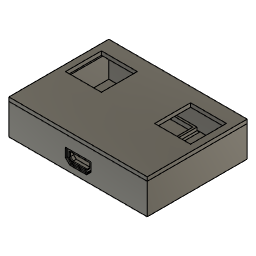
keypad_choc_white_1kgap (Autodesk Fusion 360 design; units mm, degrees)
Autodesk Fusion 360 part; units mm, degrees
sketch "Sketch1" plane through (0, 0, 0) normal (0, 0, 1) x (1, 0, 0)
  line L0 (-25, 0) -> (25, 0)
  line L1 (25, 0) -> (25, 35)
  line L2 (25, 35) -> (-25, 35)
  line L3 (-25, 35) -> (-25, 0)
  line L4 (27, -2) -> (27, 37)
  line L5 (27, 37) -> (-27, 37)
  line L6 (-27, 37) -> (-27, -2)
  line L7 (-27, -2) -> (27, -2)
  line L8 (0, 0) -> (0, -1.5)
  line L9 (-9, 0) -> (9.3, 0)
  line L10 (9.3, 0) -> (9.3, 33.5)
  line L11 (9.3, 33.5) -> (-9, 33.5)
  line L12 (-9, 33.5) -> (-9, 0)
  line L13 (-3.6938, -1.5) -> (3.8062, -1.5)
  line L14 (3.8062, -1.5) -> (3.8062, 0)
  line L15 (3.8062, 0) -> (-3.6938, 0)
  line L16 (-3.6938, 0) -> (-3.6938, -1.5)
  line L17 (10.1, 0) -> (10.1, 34.3)
  line L18 (10.1, 34.3) -> (-9.8, 34.3)
  line L19 (-9.8, 34.3) -> (-9.8, 0)
  dimension "d1" = 50
  dimension "d2" = 35
  dimension "d5" = 2
  dimension "d11" = 1.5
  dimension "d12" = 18.3
  dimension "d13" = 33.5
  dimension "d14" = 7.5
  dimension "d15" = 0.8
  constraint horizontal L0
  constraint vertical L1
  constraint horizontal L2
  constraint vertical L3
  constraint coincident L8.start origin
  constraint perpendicular L0 L8
  constraint horizontal L9
  constraint vertical L10
  constraint horizontal L11
  constraint vertical L12
  constraint coincident L0 L9.start
  constraint horizontal L13
  constraint vertical L14
  constraint horizontal L15
  constraint vertical L16
  measures "d1" distance of L0.start L0.end
  measures "d2" distance of L0.start L2.end
  measures "d11" distance of L8.start L8.end
  measures "d12" distance of L9.start L9.end
  measures "d13" distance of L9.start L11.end
  measures "d14" distance of L13.start L13.end
extrude "Extrude3" add sketch "Sketch1" along normal blind 1.7 contours L0 L10 L11 L12 L17 L18 L19 makes body 1
extrude "Extrude1" add sketch "Sketch1" against normal blind 2 separate body contours L0 L1 L2 L3 L17 L18 L19 | L0 L10 L11 L12 L17 L18 L19 | L0 L9 L10 L11 L12 L15 | L0 L8 L9 L13 L15 L16 | L0 L8 L9 L13 L14 L15 | L4 L5 L6 L7 makes body 2
extrude "Extrude2" add sketch "Sketch1" along normal blind 10 contours L0 L8 L9 L13 L15 L16 | L0 L8 L9 L13 L14 L15 | L4 L5 L6 L7 bodies 2
ref_plane "WorkPlane1" through (1.9031, -0.75, 1.7) normal (0, 0, 1) x (1, 0, 0)
sketch "Sketch2" plane through (1.9031, -0.75, 1.7) normal (0, 0, 1) x (1, 0, 0)
  line L0 (1.9031, -0.75) -> (1.9031, 0.75)
  line L1 (-5.5969, -0.75) -> (1.9031, -0.75)
  line L2 (-5.5969, 0.75) -> (-5.5969, -0.75)
  line L3 (1.9031, 0.75) -> (-5.5969, 0.75)
  line L4 (-5.5969, 0.75) -> (1.9031, 0.75)
  line L5 (1.9031, 0.75) -> (1.9031, -1.7033)
  line L6 (1.9031, -1.7033) -> (-5.5969, -1.7033)
  line L7 (-5.5969, -1.7033) -> (-5.5969, 0.75)
  constraint coincident L0.end L3.start
  constraint coincident L2.start L3.end
  constraint horizontal L4
  constraint vertical L5
  constraint horizontal L6
  constraint vertical L7
extrude "Extrude4" cut sketch "Sketch2" along normal blind 2.6 and the other way blind 0.1 bodies 2
chamfer "Chamfer1" distance 1 angle 45 2 edges at (-3.6938, -1, 1.6) (3.8062, -1, 1.6) on bodies 2
sketch "Sketch3" plane through (0, -2, 0) normal (0, -1, 0) x (1, 0, 0)
  line L0 (2.8062, 1.6) -> (-2.6938, 1.6)
  line L1 (-2.6938, 1.6) -> (-3.6938, 2.6)
  line L2 (-3.6938, 2.6) -> (-3.6938, 4.3)
  line L3 (-3.6938, 4.3) -> (3.8062, 4.3)
  line L4 (3.8062, 4.3) -> (3.8062, 2.6)
  line L5 (3.8062, 2.6) -> (2.8062, 1.6)
  line L6 (-27, 10) -> (-27, -2)
  line L7 (-27, -2) -> (27, -2)
  line L8 (27, -2) -> (27, 10)
  line L9 (27, 10) -> (-27, 10)
  line L10 (-3.6938, 4.3) -> (3.8062, 4.3)
  line L11 (3.8062, 4.3) -> (3.8062, 2.6)
  line L12 (2.8062, 1.6) -> (3.8062, 2.6)
  line L13 (2.8062, 1.6) -> (-2.6938, 1.6)
  line L14 (-3.6938, 2.6) -> (-2.6938, 1.6)
  line L15 (-3.6938, 2.6) -> (-3.6938, 4.3)
  line L16 (4.8062, 2.1858) -> (3.2204, 0.6)
  line L17 (3.2204, 0.6) -> (-3.108, 0.6)
  line L18 (-3.108, 0.6) -> (-4.6938, 2.1858)
  line L19 (-4.6938, 2.1858) -> (-4.6938, 5.3)
  line L20 (-4.6938, 5.3) -> (4.8062, 5.3)
  line L21 (4.8062, 5.3) -> (4.8062, 2.1858)
  dimension "d24" = -1
  measures "d24" distance of L5
extrude "Extrude6" cut sketch "Sketch3" against normal blind 0.5 contours L16 L17 L18 L19 L20 L21 bodies 2
fillet "Fillet1" radius 0.25 18 edges at (0.0562, -1.5, 5.3) (0.0562, -2, 5.3) (-4.6938, -1.5, 3.7429) (-4.6938, -2, 3.7429) (-3.9009, -2, 1.3929) (-3.9009, -1.5, 1.3929) (0.0562, -1.5, 0.6) (0.0562, -2, 0.6) (4.8062, -1.5, 3.7429) (4.8062, -2, 3.7429) (4.0133, -1.5, 1.3929) (4.0133, -2, 1.3929) (0.0562, -1.5, 4.3) (-3.6938, -1.5, 3.45) (-3.1938, -1.5, 2.1) (0.0562, -1.5, 1.6) (3.3062, -1.5, 2.1) (3.8062, -1.5, 3.45) on bodies 2
combine "Combine1" operation add target body 1 tool bodies 2
chamfer "Chamfer2" distance 0.5 angle 45 3 edges at (10.1, 17.15, 0) (-9.8, 17.15, 0) (0.15, 34.3, 0) on bodies 1
sketch "Sketch4" plane through (0, 0, 10) normal (0, 0, 1) x (-1, 0, 0)
  line L0 (25, 0) -> (25, -35)
  line L1 (25, -35) -> (-25, -35)
  line L2 (-25, -35) -> (-25, 0)
  line L3 (-25, 0) -> (25, 0)
  line L4 (27, 2) -> (-27, 2)
  line L5 (-27, 2) -> (-27, -37)
  line L6 (-27, -37) -> (27, -37)
  line L7 (27, -37) -> (27, 2)
  line L8 (-25, -35) -> (25, -35)
  line L9 (-25, 0) -> (-25, -35)
  line L10 (25, -35) -> (25, 0)
  line L11 (25, 0) -> (-25, 0)
  line L12 (25.8, 0.8) -> (25.8, -35.8)
  line L13 (25.8, -35.8) -> (-25.8, -35.8)
  line L14 (-25.8, -35.8) -> (-25.8, 0.8)
  line L15 (-25.8, 0.8) -> (25.8, 0.8)
  dimension "d32" = -0.8
extrude "Extrude7" cut sketch "Sketch4" against normal blind 1 contours L12 L13 L14 L15 bodies 1
sketch "Sketch5" plane through (0, 0, 9) normal (0, 0, 1) x (-1, 0, 0)
  line L0 (-25, 0) -> (25, 0)
  line L1 (25, 0) -> (25, -35)
  line L2 (25, -35) -> (-25, -35)
  line L3 (-25, -35) -> (-25, 0)
  line L4 (-25.8, 0.8) -> (-25.8, -35.8)
  line L5 (-25.8, -35.8) -> (25.8, -35.8)
  line L6 (25.8, -35.8) -> (25.8, 0.8)
  line L7 (25.8, 0.8) -> (-25.8, 0.8)
  line L8 (-25.8, -35.8) -> (-25.8, 0.8)
  line L9 (25.8, -35.8) -> (-25.8, -35.8)
  line L10 (25.8, 0.8) -> (25.8, -35.8)
  line L11 (-25.8, 0.8) -> (25.8, 0.8)
  line L12 (25.6, -35.6) -> (25.6, 0.6)
  line L13 (25.6, 0.6) -> (-25.6, 0.6)
  line L14 (-25.6, 0.6) -> (-25.6, -35.6)
  line L15 (-25.6, -35.6) -> (25.6, -35.6)
  dimension "d35" = -0.2
extrude "Extrude8" add sketch "Sketch5" along normal blind 1 separate body contours L12 L13 L14 L15 makes body 3
sketch "Sketch6" plane through (0, 0, 10) normal (0, 0, 1) x (-1, 0, 0)
  line L0 (25, -35) -> (-25, -35)
  line L1 (-25, -35) -> (-25, 0)
  line L2 (-25, 0) -> (25, 0)
  line L3 (25, 0) -> (25, -35)
  line L4 (-25.6, -35.6) -> (25.6, -35.6)
  line L5 (25.6, -35.6) -> (25.6, 0.6)
  line L6 (25.6, 0.6) -> (-25.6, 0.6)
  line L7 (-25.6, 0.6) -> (-25.6, -35.6)
  line L8 (27, -37) -> (-27, -37)
  line L9 (-27, -37) -> (-27, 2)
  line L10 (-27, 2) -> (27, 2)
  line L11 (27, 2) -> (27, -37)
  constraint horizontal L8
  constraint vertical L9
  constraint horizontal L10
  constraint vertical L11
extrude "Extrude9" add sketch "Sketch6" along normal blind 1.5 separate body contours L0 L1 L2 L3 | L4 L5 L6 L7 | L8 L9 L10 L11 makes body 4
combine "Combine2" operation add target body 4 tool bodies 3
sketch "Sketch7" plane through (0, 0, 11.5) normal (0, 0, 1) x (-1, 0, 0)
  line L0 (27, 2) -> (-27, 2)
  line L1 (-27, 2) -> (-27, -37)
  line L2 (-27, -37) -> (27, -37)
  line L3 (27, -37) -> (27, 2)
  line L4 (24.514, -17.628) -> (10.514, -17.628)
  line L5 (10.514, -17.628) -> (10.514, -31.628)
  line L6 (10.514, -31.628) -> (24.514, -31.628)
  line L7 (24.514, -31.628) -> (24.514, -17.628)
  line L8 (-24.4142, -17.48) -> (-24.4142, -31.48)
  line L9 (-24.4142, -31.48) -> (-10.4142, -31.48)
  line L10 (-10.4142, -31.48) -> (-10.4142, -17.48)
  line L11 (-10.4142, -17.48) -> (-24.4142, -17.48)
  dimension "d40" = 14
  dimension "d41" = 14
  dimension "d42" = 14
  dimension "d43" = 14
  constraint horizontal L4
  constraint vertical L5
  constraint horizontal L6
  constraint vertical L7
  constraint horizontal L11
  constraint vertical L8
  constraint horizontal L9
  constraint vertical L10
  measures "d40" distance of L4.start L4.end
  measures "d41" distance of L4.start L6.end
  measures "d42" distance of L8.start L10.end
  measures "d43" distance of L9.end L10.end
extrude "Extrude10" cut sketch "Sketch7" against normal blind 3 contours L4 L5 L6 L7 | L8 L9 L10 L11 bodies 4
